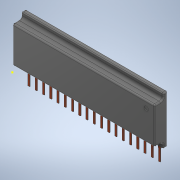
# Autodesk Inventor part: КХА058
Saved by Autodesk Inventor 2020.2 (Build 242310000, 310)
## iProperties
Created: 2020-03-30
Part Number: КХА058
Material: Generic
Document SubType Name: Modeling
Designer: IAmIllusion
Density: 1 g/cm^3
Appearance: Default
Author: IAmIllusion
Autodesk Inventor part; units mm, degrees
ref_plane "YZ Plane" through (0, 0, 0) normal (1, 0, 0) x (0, 1, 0)
ref_plane "XZ Plane" through (0, 0, 0) normal (0, 1, 0) x (-1, 0, 0)
ref_plane "XY Plane" through (0, 0, 0) normal (0, 0, 1) x (1, 0, 0)
sketch "Sketch1" plane through (0, 0, 0) normal (1, 0, 0) x (0, 1, 0)
  line L0 (0.3, 0) -> (16.325, 0)
  line L1 (16.625, 0.3) -> (16.625, 1.2)
  line L2 (0, 1.2) -> (0, 0.3)
  line L3 (14.625, 2.5) -> (14.625, 4)
  line L4 (14.125, 4.5) -> (2.5, 4.5)
  line L5 (2, 4) -> (2, 2.5)
  line L6 (16.325, 1.5) -> (15.625, 1.5)
  line L7 (0.3, 1.5) -> (1, 1.5)
  arc A0 (14.625, 4) -> (14.125, 4.5) centre (14.125, 4) ccw
  arc A1 (2.5, 4.5) -> (2, 4) centre (2.5, 4) ccw
  arc A2 (14.625, 2.5) -> (15.625, 1.5) centre (15.625, 2.5) ccw
  arc A3 (1, 1.5) -> (2, 2.5) centre (1, 2.5) ccw
  line L8 (15.625, 1.5) -> (1, 1.5)
  arc A4 (16.625, 1.2) -> (16.325, 1.5) centre (16.325, 1.2) ccw
  arc A5 (16.325, 0) -> (16.625, 0.3) centre (16.325, 0.3) ccw
  arc A6 (0.3, 1.5) -> (0, 1.2) centre (0.3, 1.2) ccw
  arc A7 (0, 0.3) -> (0.3, 0) centre (0.3, 0.3) ccw
  point P0 (0, 0)
  constraints: 18 end point, 17 tangent, 16 point on circle, 8 centre point, 4 equal radius, 4 horizontal, 2 point on line, 1 collinear, 1 parallel, 1 perpendicular, 1 vertical
extrude "Extrusion1" add sketch "Sketch1" along normal blind 49
sketch "Sketch2" plane through (0, 0, 0.3) normal (0, -1, 0) x (1, 0, 0)
  line L0 (0, 0) -> (0, 0.9) projected
  line L1 (0, 0.9) -> (49, 0.9) projected
  line L2 (0, 0.45) -> (2, 0.45)
  line L3 (2, 0.45) -> (4.5, 0.45)
  line L4 (4.5, 0.45) -> (7, 0.45)
  line L5 (7, 0.45) -> (9.5, 0.45)
  line L6 (9.5, 0.45) -> (12, 0.45)
  line L7 (12, 0.45) -> (14.5, 0.45)
  line L8 (14.5, 0.45) -> (17, 0.45)
  line L9 (17, 0.45) -> (19.5, 0.45)
  line L10 (19.5, 0.45) -> (22, 0.45)
  line L11 (22, 0.45) -> (24.5, 0.45)
  line L12 (24.5, 0.45) -> (27, 0.45)
  line L13 (27, 0.45) -> (29.5, 0.45)
  line L14 (29.5, 0.45) -> (32, 0.45)
  line L15 (32, 0.45) -> (34.5, 0.45)
  line L16 (34.5, 0.45) -> (37, 0.45)
  line L17 (37, 0.45) -> (39.5, 0.45)
  line L18 (39.5, 0.45) -> (42, 0.45)
  line L19 (42, 0.45) -> (44.5, 0.45)
  line L20 (44.5, 0.45) -> (47, 0.45)
  line L21 (47, 0.45) -> (49, 0.45)
  line L22 (49, -0.3) -> (49, 0) projected
  line L23 (2, 0.45) -> (1.6, 0.45)
  line L24 (1.6, 0.45) -> (1.6, 0.575)
  line L25 (1.6, 0.575) -> (2.4, 0.575)
  line L26 (2.4, 0.575) -> (2.4, 0.325)
  line L27 (2.4, 0.325) -> (1.6, 0.325)
  line L28 (1.6, 0.325) -> (1.6, 0.45)
  line L29 (4.5, 0.45) -> (4.1, 0.45)
  line L30 (4.1, 0.45) -> (4.1, 0.575)
  line L31 (4.1, 0.575) -> (4.9, 0.575)
  line L32 (4.9, 0.575) -> (4.9, 0.325)
  line L33 (4.9, 0.325) -> (4.1, 0.325)
  line L34 (4.1, 0.325) -> (4.1, 0.45)
  line L35 (7, 0.45) -> (6.6, 0.45)
  line L36 (6.6, 0.45) -> (6.6, 0.575)
  line L37 (6.6, 0.575) -> (7.4, 0.575)
  line L38 (7.4, 0.575) -> (7.4, 0.325)
  line L39 (7.4, 0.325) -> (6.6, 0.325)
  line L40 (6.6, 0.325) -> (6.6, 0.45)
  line L41 (9.5, 0.45) -> (9.1, 0.45)
  line L42 (9.1, 0.45) -> (9.1, 0.575)
  line L43 (9.1, 0.575) -> (9.9, 0.575)
  line L44 (9.9, 0.575) -> (9.9, 0.325)
  line L45 (9.9, 0.325) -> (9.1, 0.325)
  line L46 (9.1, 0.325) -> (9.1, 0.45)
  line L47 (12, 0.45) -> (11.6, 0.45)
  line L48 (11.6, 0.45) -> (11.6, 0.575)
  line L49 (11.6, 0.575) -> (12.4, 0.575)
  line L50 (12.4, 0.575) -> (12.4, 0.325)
  line L51 (12.4, 0.325) -> (11.6, 0.325)
  line L52 (11.6, 0.325) -> (11.6, 0.45)
  line L53 (14.5, 0.45) -> (14.1, 0.45)
  line L54 (14.1, 0.45) -> (14.1, 0.575)
  line L55 (14.1, 0.575) -> (14.9, 0.575)
  line L56 (14.9, 0.575) -> (14.9, 0.325)
  line L57 (14.9, 0.325) -> (14.1, 0.325)
  line L58 (14.1, 0.325) -> (14.1, 0.45)
  line L59 (17, 0.45) -> (16.6, 0.45)
  line L60 (16.6, 0.45) -> (16.6, 0.575)
  line L61 (16.6, 0.575) -> (17.4, 0.575)
  line L62 (17.4, 0.575) -> (17.4, 0.325)
  line L63 (17.4, 0.325) -> (16.6, 0.325)
  line L64 (16.6, 0.325) -> (16.6, 0.45)
  line L65 (19.5, 0.45) -> (19.1, 0.45)
  line L66 (19.1, 0.45) -> (19.1, 0.575)
  line L67 (19.1, 0.575) -> (19.9, 0.575)
  line L68 (19.9, 0.575) -> (19.9, 0.325)
  line L69 (19.9, 0.325) -> (19.1, 0.325)
  line L70 (19.1, 0.325) -> (19.1, 0.45)
  line L71 (22, 0.45) -> (21.6, 0.45)
  line L72 (21.6, 0.45) -> (21.6, 0.575)
  line L73 (21.6, 0.575) -> (22.4, 0.575)
  line L74 (22.4, 0.575) -> (22.4, 0.325)
  line L75 (22.4, 0.325) -> (21.6, 0.325)
  line L76 (21.6, 0.325) -> (21.6, 0.45)
  line L77 (24.5, 0.45) -> (24.1, 0.45)
  line L78 (24.1, 0.45) -> (24.1, 0.575)
  line L79 (24.1, 0.575) -> (24.9, 0.575)
  line L80 (24.9, 0.575) -> (24.9, 0.325)
  line L81 (24.9, 0.325) -> (24.1, 0.325)
  line L82 (24.1, 0.325) -> (24.1, 0.45)
  line L83 (27, 0.45) -> (26.6, 0.45)
  line L84 (26.6, 0.45) -> (26.6, 0.575)
  line L85 (26.6, 0.575) -> (27.4, 0.575)
  line L86 (27.4, 0.575) -> (27.4, 0.325)
  line L87 (27.4, 0.325) -> (26.6, 0.325)
  line L88 (26.6, 0.325) -> (26.6, 0.45)
  line L89 (29.5, 0.45) -> (29.1, 0.45)
  line L90 (29.1, 0.45) -> (29.1, 0.575)
  line L91 (29.1, 0.575) -> (29.9, 0.575)
  line L92 (29.9, 0.575) -> (29.9, 0.325)
  line L93 (29.9, 0.325) -> (29.1, 0.325)
  line L94 (29.1, 0.325) -> (29.1, 0.45)
  line L95 (32, 0.45) -> (31.6, 0.45)
  line L96 (31.6, 0.45) -> (31.6, 0.575)
  line L97 (31.6, 0.575) -> (32.4, 0.575)
  line L98 (32.4, 0.575) -> (32.4, 0.325)
  line L99 (32.4, 0.325) -> (31.6, 0.325)
  line L100 (31.6, 0.325) -> (31.6, 0.45)
  line L101 (34.5, 0.45) -> (34.1, 0.45)
  line L102 (34.1, 0.45) -> (34.1, 0.575)
  line L103 (34.1, 0.575) -> (34.9, 0.575)
  line L104 (34.9, 0.575) -> (34.9, 0.325)
  line L105 (34.9, 0.325) -> (34.1, 0.325)
  line L106 (34.1, 0.325) -> (34.1, 0.45)
  line L107 (37, 0.45) -> (36.6, 0.45)
  line L108 (36.6, 0.45) -> (36.6, 0.575)
  line L109 (36.6, 0.575) -> (37.4, 0.575)
  line L110 (37.4, 0.575) -> (37.4, 0.325)
  line L111 (37.4, 0.325) -> (36.6, 0.325)
  line L112 (36.6, 0.325) -> (36.6, 0.45)
  line L113 (39.5, 0.45) -> (39.1, 0.45)
  line L114 (39.1, 0.45) -> (39.1, 0.575)
  line L115 (39.1, 0.575) -> (39.9, 0.575)
  line L116 (39.9, 0.575) -> (39.9, 0.325)
  line L117 (39.9, 0.325) -> (39.1, 0.325)
  line L118 (39.1, 0.325) -> (39.1, 0.45)
  line L119 (42, 0.45) -> (41.6, 0.45)
  line L120 (41.6, 0.45) -> (41.6, 0.575)
  line L121 (41.6, 0.575) -> (42.4, 0.575)
  line L122 (42.4, 0.575) -> (42.4, 0.325)
  line L123 (42.4, 0.325) -> (41.6, 0.325)
  line L124 (41.6, 0.325) -> (41.6, 0.45)
  line L125 (44.5, 0.45) -> (44.1, 0.45)
  line L126 (44.1, 0.45) -> (44.1, 0.575)
  line L127 (44.1, 0.575) -> (44.9, 0.575)
  line L128 (44.9, 0.575) -> (44.9, 0.325)
  line L129 (44.9, 0.325) -> (44.1, 0.325)
  line L130 (44.1, 0.325) -> (44.1, 0.45)
  line L131 (47, 0.45) -> (46.6, 0.45)
  line L132 (46.6, 0.45) -> (46.6, 0.575)
  line L133 (46.6, 0.575) -> (47.4, 0.575)
  line L134 (47.4, 0.575) -> (47.4, 0.325)
  line L135 (47.4, 0.325) -> (46.6, 0.325)
  line L136 (46.6, 0.325) -> (46.6, 0.45)
  point P0 (0, -0.3)
  dimension "d24" = 2.5
  dimension "d25" = 2.5
  dimension "d26" = 2.5
  dimension "d27" = 2.5
  dimension "d28" = 2.5
  dimension "d29" = 2.5
  dimension "d30" = 2.5
  dimension "d31" = 2.5
  dimension "d32" = 2.5
  dimension "d33" = 2.5
  dimension "d34" = 2.5
  dimension "d35" = 2.5
  dimension "d36" = 2.5
  dimension "d37" = 2.5
  dimension "d38" = 2.5
  dimension "d39" = 2.5
  dimension "d40" = 2.5
  dimension "d41" = 2.5
  constraints: 268 end point, 93 perpendicular, 56 point on line, 1 horizontal, 1 midpoint
  measures "d24" distance of L2.end L3.end
  measures "d25" distance of L3.end L4.end
  measures "d26" distance of L4.end L5.end
  measures "d27" distance of L5.end L6.end
  measures "d28" distance of L6.end L7.end
  measures "d29" distance of L7.end L8.end
  measures "d30" distance of L8.end L9.end
  measures "d31" distance of L9.end L10.end
  measures "d32" distance of L10.end L11.end
  measures "d33" distance of L11.end L12.end
  measures "d34" distance of L12.end L13.end
  measures "d35" distance of L13.end L14.end
  measures "d36" distance of L14.end L15.end
  measures "d37" distance of L15.end L16.end
  measures "d38" distance of L16.end L17.end
  measures "d39" distance of L17.end L18.end
  measures "d40" distance of L18.end L19.end
  measures "d41" distance of L19.end L20.end
extrude "Extrusion2" add sketch "Sketch2" along normal blind 1
sketch "Sketch3" plane through (0, -1, 0.3) normal (0, -1, 0) x (1, 0, 0)
  line L0 (1.6, 0.325) -> (1.6, 0.575) projected
  line L1 (2.4, 0.575) -> (1.6, 0.575) projected
  line L2 (1.7, 0.575) -> (1.7, 0.325)
  line L3 (1.6, 0.325) -> (2.4, 0.325) projected
  line L4 (1.7, 0.575) -> (2.3, 0.575)
  line L5 (2.3, 0.575) -> (2.3, 0.325)
  point P0 (0, -0.3)
  constraints: 6 end point, 4 point on line, 1 perpendicular
extrude "Extrusion3" add sketch "Sketch3" along normal blind 4 contours L2 L1 L5 L3
chamfer "Chamfer1" distance 0.1 angle 45 1 edges at (2.4, -1, 0.75)
chamfer "Chamfer2" distance 0.1 angle 45 1 edges at (1.6, -1, 0.75)
sketch "Sketch4" plane through (0, -1, 0.3) normal (0, -1, 0) x (1, 0, 0)
  line L0 (4.1, 0.325) -> (4.1, 0.575) projected
  line L1 (4.1, 0.575) -> (4.2, 0.575)
  line L2 (4.9, 0.575) -> (4.1, 0.575) projected
  line L3 (4.2, 0.575) -> (4.2, 0.325)
  line L4 (4.2, 0.325) -> (4.8, 0.325)
  line L5 (4.1, 0.325) -> (4.9, 0.325) projected
  line L6 (4.8, 0.325) -> (4.8, 0.575)
  line L7 (4.8, 0.575) -> (4.2, 0.575)
  point P0 (0, -0.3)
  constraints: 10 end point, 3 point on line, 1 collinear, 1 perpendicular
extrude "Extrusion4" add sketch "Sketch4" along normal blind 4 contours L3 L2 L6 L4
sketch "Sketch5" plane through (0, -1, 0.3) normal (0, -1, 0) x (1, 0, 0)
  line L0 (6.6, 0.575) -> (6.7, 0.575)
  line L1 (7.4, 0.575) -> (6.6, 0.575) projected
  line L2 (6.7, 0.575) -> (6.7, 0.325)
  line L3 (6.7, 0.325) -> (7.3, 0.325)
  line L4 (6.6, 0.325) -> (7.4, 0.325) projected
  line L5 (7.3, 0.325) -> (7.3, 0.575)
  point P0 (0, -0.3)
  constraints: 8 end point, 3 point on line, 2 perpendicular
extrude "Extrusion5" add sketch "Sketch5" along normal blind 4
sketch "Sketch6" plane through (0, -1, 0.3) normal (0, -1, 0) x (1, 0, 0)
  line L0 (9.1, 0.575) -> (9.1, 0.325) projected
  line L1 (9.1, 0.575) -> (9.2, 0.575)
  line L2 (9.9, 0.575) -> (9.1, 0.575) projected
  line L3 (9.2, 0.575) -> (9.2, 0.325)
  line L4 (9.2, 0.325) -> (9.8, 0.325)
  line L5 (9.1, 0.325) -> (9.9, 0.325) projected
  line L6 (9.8, 0.325) -> (9.8, 0.575)
  line L7 (12.4, 0.575) -> (11.6, 0.575) projected
  line L8 (11.6, 0.575) -> (11.7, 0.575)
  line L9 (11.7, 0.575) -> (11.7, 0.325)
  line L10 (11.7, 0.325) -> (12.3, 0.325)
  line L11 (12.4, 0.325) -> (11.6, 0.325) projected
  line L12 (12.3, 0.325) -> (12.3, 0.575)
  line L13 (14.9, 0.575) -> (14.1, 0.575) projected
  line L14 (14.1, 0.575) -> (14.2, 0.575)
  line L15 (14.2, 0.575) -> (14.2, 0.325)
  line L16 (14.1, 0.325) -> (14.9, 0.325) projected
  line L17 (14.2, 0.325) -> (14.8, 0.325)
  line L18 (14.8, 0.325) -> (14.8, 0.575)
  line L19 (17.4, 0.575) -> (16.6, 0.575) projected
  line L20 (16.6, 0.575) -> (16.7, 0.575)
  line L21 (16.7, 0.575) -> (16.7, 0.325)
  line L22 (16.7, 0.325) -> (17.3, 0.325)
  line L23 (16.6, 0.325) -> (17.4, 0.325) projected
  line L24 (17.3, 0.325) -> (17.3, 0.575)
  line L25 (19.9, 0.575) -> (19.1, 0.575) projected
  line L26 (19.1, 0.575) -> (19.2, 0.575)
  line L27 (19.2, 0.575) -> (19.2, 0.325)
  line L28 (19.2, 0.325) -> (19.8, 0.325)
  line L29 (19.1, 0.325) -> (19.9, 0.325) projected
  line L30 (19.8, 0.325) -> (19.8, 0.575)
  line L31 (19.8, 0.575) -> (19.2, 0.575)
  line L32 (21.6, 0.325) -> (21.6, 0.575) projected
  line L33 (21.6, 0.575) -> (21.7, 0.575)
  line L34 (21.6, 0.575) -> (22.4, 0.575) projected
  line L35 (21.7, 0.575) -> (21.7, 0.325)
  line L36 (21.7, 0.325) -> (22.3, 0.325)
  line L37 (21.6, 0.325) -> (22.4, 0.325) projected
  line L38 (22.3, 0.325) -> (22.3, 0.575)
  line L39 (22.3, 0.575) -> (21.7, 0.575)
  line L40 (24.9, 0.575) -> (24.1, 0.575) projected
  line L41 (24.1, 0.575) -> (24.2, 0.575)
  line L42 (24.2, 0.575) -> (24.2, 0.325)
  line L43 (24.2, 0.325) -> (24.8, 0.325)
  line L44 (24.1, 0.325) -> (24.9, 0.325) projected
  line L45 (24.8, 0.325) -> (24.8, 0.575)
  line L46 (26.6, 0.325) -> (26.6, 0.575) projected
  line L47 (26.6, 0.575) -> (26.7, 0.575)
  line L48 (27.4, 0.575) -> (26.6, 0.575) projected
  line L49 (26.7, 0.575) -> (26.7, 0.325)
  line L50 (26.6, 0.325) -> (27.4, 0.325) projected
  line L51 (26.7, 0.325) -> (27.3, 0.325)
  line L52 (27.3, 0.325) -> (27.3, 0.575)
  line L53 (29.1, 0.575) -> (29.1, 0.325) projected
  line L54 (29.1, 0.575) -> (29.2, 0.575)
  line L55 (29.9, 0.575) -> (29.1, 0.575) projected
  line L56 (29.2, 0.575) -> (29.2, 0.325)
  line L57 (29.9, 0.325) -> (29.1, 0.325) projected
  line L58 (29.2, 0.325) -> (29.8, 0.325)
  line L59 (29.8, 0.325) -> (29.8, 0.575)
  line L60 (31.6, 0.575) -> (32.4, 0.575) projected
  line L61 (31.6, 0.575) -> (31.7, 0.575)
  line L62 (31.7, 0.575) -> (31.7, 0.325)
  line L63 (32.4, 0.325) -> (31.6, 0.325) projected
  line L64 (31.7, 0.325) -> (32.3, 0.325)
  line L65 (32.3, 0.325) -> (32.3, 0.575)
  line L66 (32.3, 0.575) -> (31.7, 0.575)
  line L67 (34.1, 0.575) -> (34.1, 0.325) projected
  line L68 (34.1, 0.575) -> (34.2, 0.575)
  line L69 (34.9, 0.575) -> (34.1, 0.575) projected
  line L70 (34.2, 0.575) -> (34.2, 0.325)
  line L71 (34.2, 0.325) -> (34.8, 0.325)
  line L72 (34.1, 0.325) -> (34.9, 0.325) projected
  line L73 (34.8, 0.325) -> (34.8, 0.575)
  line L74 (34.8, 0.575) -> (34.2, 0.575)
  line L75 (36.6, 0.575) -> (36.6, 0.325) projected
  line L76 (36.6, 0.575) -> (36.7, 0.575)
  line L77 (36.6, 0.575) -> (37.4, 0.575) projected
  line L78 (36.7, 0.575) -> (36.7, 0.325)
  line L79 (36.7, 0.325) -> (37.3, 0.325)
  line L80 (36.6, 0.325) -> (37.4, 0.325) projected
  line L81 (37.3, 0.325) -> (37.3, 0.575)
  line L82 (39.9, 0.575) -> (39.1, 0.575) projected
  line L83 (39.1, 0.575) -> (39.2, 0.575)
  line L84 (39.2, 0.575) -> (39.2, 0.325)
  line L85 (39.2, 0.325) -> (39.8, 0.325)
  line L86 (39.1, 0.325) -> (39.9, 0.325) projected
  line L87 (39.8, 0.325) -> (39.8, 0.575)
  line L88 (39.8, 0.575) -> (39.2, 0.575)
  line L89 (41.6, 0.575) -> (41.6, 0.325) projected
  line L90 (41.6, 0.575) -> (41.7, 0.575)
  line L91 (42.4, 0.575) -> (41.6, 0.575) projected
  line L92 (41.7, 0.575) -> (41.7, 0.325)
  line L93 (41.7, 0.325) -> (42.3, 0.325)
  line L94 (41.6, 0.325) -> (42.4, 0.325) projected
  line L95 (42.3, 0.325) -> (42.3, 0.575)
  line L96 (42.3, 0.575) -> (41.7, 0.575)
  line L97 (44.1, 0.575) -> (44.1, 0.325) projected
  line L98 (44.1, 0.575) -> (44.2, 0.575)
  line L99 (44.1, 0.575) -> (44.9, 0.575) projected
  line L100 (44.2, 0.575) -> (44.2, 0.325)
  line L101 (44.2, 0.325) -> (44.8, 0.325)
  line L102 (44.1, 0.325) -> (44.9, 0.325) projected
  line L103 (44.8, 0.325) -> (44.8, 0.575)
  line L104 (44.8, 0.575) -> (44.2, 0.575)
  line L105 (47.4, 0.575) -> (46.6, 0.575) projected
  line L106 (46.6, 0.575) -> (46.7, 0.575)
  line L107 (46.7, 0.575) -> (46.7, 0.325)
  line L108 (46.7, 0.325) -> (47.3, 0.325)
  line L109 (47.4, 0.325) -> (46.6, 0.325) projected
  line L110 (47.3, 0.325) -> (47.3, 0.575)
  line L111 (47.3, 0.575) -> (46.7, 0.575)
  point P0 (0, -0.3)
  point P1 (39.8, 0.575)
  point P2 (34.8, 0.575)
  point P3 (32.3, 0.325)
  point P4 (32.3, 0.575)
  point P5 (22.3, 0.575)
  constraints: 144 end point, 51 point on line, 28 perpendicular, 2 collinear, 2 vertical
extrude "Extrusion6" add sketch "Sketch6" along normal blind 4 contours L2 L6 L4 L3 | L12 L10 L9 L7 | L18 L16 L15 L13 | L24 L22 L21 L19 | L30 L28 L27 L25 | L35 L34 L38 L36 | L45 L43 L42 L40 | L49 L48 L52 L50 | L55 L59 L57 L56 | L60 L65 L63 L62 | L69 L73 L71 L70 | L77 L81 L79 L78 | L87 L85 L84 L82 | L91 L95 L93 L92 | L99 L103 L101 L100 | L110 L108 L107 L105
chamfer "Chamfer3" distance 0.1 angle 45 1 edges at (4.1, -1, 0.75)
chamfer "Chamfer4" distance 0.1 angle 45 1 edges at (4.9, -1, 0.75)
chamfer "Chamfer5" distance 0.1 angle 45 1 edges at (6.6, -1, 0.75)
chamfer "Chamfer6" distance 0.1 angle 45 1 edges at (7.4, -1, 0.75)
chamfer "Chamfer7" distance 0.1 angle 45 1 edges at (9.1, -1, 0.75)
chamfer "Chamfer8" distance 0.1 angle 45 1 edges at (9.9, -1, 0.75)
chamfer "Chamfer9" distance 0.1 angle 45 1 edges at (11.6, -1, 0.75)
chamfer "Chamfer10" distance 0.1 angle 45 1 edges at (12.4, -1, 0.75)
chamfer "Chamfer11" distance 0.1 angle 45 1 edges at (14.1, -1, 0.75)
chamfer "Chamfer12" distance 0.1 angle 45 1 edges at (14.9, -1, 0.75)
chamfer "Chamfer13" distance 0.1 angle 45 1 edges at (16.6, -1, 0.75)
chamfer "Chamfer14" distance 0.1 angle 45 1 edges at (17.4, -1, 0.75)
chamfer "Chamfer15" distance 0.1 angle 45 1 edges at (19.1, -1, 0.75)
chamfer "Chamfer16" distance 0.1 angle 45 1 edges at (19.9, -1, 0.75)
chamfer "Chamfer17" distance 0.1 angle 45 1 edges at (21.6, -1, 0.75)
chamfer "Chamfer18" distance 0.1 angle 45 1 edges at (22.4, -1, 0.75)
chamfer "Chamfer19" distance 0.1 angle 45 1 edges at (24.1, -1, 0.75)
chamfer "Chamfer20" distance 0.1 angle 45 1 edges at (24.9, -1, 0.75)
chamfer "Chamfer21" distance 0.1 angle 45 1 edges at (26.6, -1, 0.75)
chamfer "Chamfer22" distance 0.1 angle 45 1 edges at (27.4, -1, 0.75)
chamfer "Chamfer23" distance 0.1 angle 45 1 edges at (29.1, -1, 0.75)
chamfer "Chamfer24" distance 0.1 angle 45 1 edges at (29.9, -1, 0.75)
chamfer "Chamfer25" distance 0.1 angle 45 1 edges at (31.6, -1, 0.75)
chamfer "Chamfer26" distance 0.1 angle 45 1 edges at (32.4, -1, 0.75)
chamfer "Chamfer27" distance 0.1 angle 45 1 edges at (34.1, -1, 0.75)
chamfer "Chamfer28" distance 0.1 angle 45 1 edges at (34.9, -1, 0.75)
chamfer "Chamfer29" distance 0.1 angle 45 1 edges at (36.6, -1, 0.75)
chamfer "Chamfer30" distance 0.1 angle 45 1 edges at (37.4, -1, 0.75)
chamfer "Chamfer31" distance 0.1 angle 45 1 edges at (39.1, -1, 0.75)
chamfer "Chamfer32" distance 0.1 angle 45 1 edges at (39.9, -1, 0.75)
chamfer "Chamfer33" distance 0.1 angle 45 1 edges at (41.6, -1, 0.75)
chamfer "Chamfer34" distance 0.1 angle 45 1 edges at (42.4, -1, 0.75)
chamfer "Chamfer35" distance 0.1 angle 45 1 edges at (44.1, -1, 0.75)
chamfer "Chamfer36" distance 0.1 angle 45 1 edges at (44.9, -1, 0.75)
chamfer "Chamfer37" distance 0.1 angle 45 1 edges at (46.6, -1, 0.75)
chamfer "Chamfer38" distance 0.1 angle 45 1 edges at (47.4, -1, 0.75)
sketch "Sketch7" plane through (0, 2.5, 4.5) normal (0, 0, 1) x (1, 0, 0)
  point P0 (0, -2.5)
sketch "Sketch8" plane through (0, 2.5, 4.5) normal (0, 0, 1) x (1, 0, 0)
  circle A0 centre (46.1772, 9.7786) radius 0.75
  point P0 (0, -2.5)
  constraints: 1 centre point
extrude "Extrusion7" cut sketch "Sketch8" against normal blind 0.2
fillet "Fillet1" radius 0.5 16 edges at (0, 2.1464, 4.3536) (0, 2, 3.25) (0, 1.7071, 1.7929) (0, 0.65, 1.5) (0, 0.0879, 1.4121) (0, 0, 0.75) (0, 0.0879, 0.0879) (0, 8.3125, 0) (0, 16.5371, 0.0879) (0, 16.625, 0.75) (0, 16.5371, 1.4121) (0, 15.975, 1.5) (0, 14.9179, 1.7929) (0, 14.625, 3.25) (0, 14.4786, 4.3536) (0, 8.3125, 4.5)
fillet "Fillet2" radius 0.5 16 edges at (49, 16.5371, 0.0879) (49, 16.625, 0.75) (49, 16.5371, 1.4121) (49, 15.975, 1.5) (49, 14.9179, 1.7929) (49, 14.625, 3.25) (49, 14.4786, 4.3536) (49, 8.3125, 4.5) (49, 2.1464, 4.3536) (49, 2, 3.25) (49, 1.7071, 1.7929) (49, 0.65, 1.5) (49, 0.0879, 1.4121) (49, 0, 0.75) (49, 0.0879, 0.0879) (49, 8.3125, 0)
body "Solid1"
